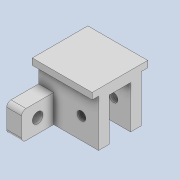
# Autodesk Inventor part: 10-03-025
Saved by Autodesk Inventor 2020 (Build 240168000, 168)
## iProperties
Created: 2019-11-02
Part Number: 10-03-025
Material: Generic
Document SubType Name: Modeling
Designer: iuliu
Density: 1 g/cm^3
Appearance: Default
Description: Intinzator Y
Mass: 10.4136 g
Surface Area: 53.1849 cm^2
Volume: 10.4136 cm^3
Author: iuliu
Subject: 036
Autodesk Inventor part; units mm, degrees
ref_plane "YZ Plane" through (0, 0, 0) normal (1, 0, 0) x (0, 1, 0)
ref_plane "XZ Plane" through (0, 0, 0) normal (0, 1, 0) x (-1, 0, 0)
ref_plane "XY Plane" through (0, 0, 0) normal (0, 0, 1) x (1, 0, 0)
sketch "Sketch7" plane through (0, 0, 0) normal (1, 0, 0) x (0, 0, -1)
  line L0 (10, -2.5) -> (-10, -2.5)
  line L1 (-10, -2.5) -> (-10, 22.5)
  line L2 (-10, 22.5) -> (10, 22.5)
  line L3 (10, 22.5) -> (10, -2.5)
  line L4 (13, 19.5) -> (10, 19.5)
  line L5 (10, 19.5) -> (10, 22.5)
  line L6 (10, 22.5) -> (13, 22.5)
  line L7 (13, 22.5) -> (13, 19.5)
  line L8 (-10, 19.5) -> (-13, 19.5)
  line L9 (-13, 19.5) -> (-13, 22.5)
  line L10 (-13, 22.5) -> (-10, 22.5)
  line L11 (-10, 22.5) -> (-10, 19.5)
  point P0 (0, -2.5)
  point P1 (0, 22.5)
  dimension "d26" = 20
  dimension "d27" = 25
  dimension "d30" = 3
  dimension "d31" = 3
  dimension "d32" = 3
  dimension "d33" = 3
  dimension "d72" = 0
  constraints: 24 end point, 6 parallel, 3 horizontal, 3 perpendicular, 1 collinear, 1 midpoint, 1 point on line
  measures "d26" distance between parallel lines of L1 L3
  measures "d27" distance of L2.end L0.start
  measures "d30" distance of L6.end L4.start
  measures "d31" distance of L4.start L4.end
  measures "d32" distance of L8.start L8.end
  measures "d33" distance of L8.end L9.end
  measures "d72" distance from line of point (0, -2.5) L0
extrude "Extrusion4" add sketch "Sketch7" along normal blind 28
sketch "Sketch15" plane through (0, -2.5, -10) normal (0, 0, -1) x (-1, 0, 0)
  line L0 (0, 0) -> (-28, 0) projected
  line L1 (-28, 0) -> (-28, 22) projected
  point P0 (0, 2.5)
  point P1 (-20, 10)
  dimension "d78" = 8
  dimension "d98" = 10
  measures "d78" distance from line of L1 point (-20, 10)
  measures "d98" distance from line of L0 point (-20, 10)
sketch "Sketch14" plane through (0, -2.5, -10) normal (0, -1, 0) x (1, 0, 0)
  line L0 (7, 15) -> (28, 15)
  line L1 (28, 15) -> (28, 5)
  line L2 (28, 5) -> (7, 5)
  line L3 (7, 5) -> (7, 15)
  line L4 (28, 20) -> (28, 0) projected
  point P0 (0, 10)
  point P1 (28, 10)
  point P2 (28, 10)
  dimension "d73" = 10
  dimension "d74" = 21
  constraints: 8 end point, 2 midpoint, 2 parallel, 1 coincident, 1 collinear, 1 horizontal, 1 perpendicular
  measures "d73" distance of L0.end L1.end
  measures "d74" distance of L0.start L0.end
extrude "Extrusion8" cut sketch "Sketch14" against normal blind 20
hole "Hole6" at (20, 7.5, -10) direction (0, 0, 1) diameter 4.134 end through all thread size "M5x0.8" class "6H" standard "ISO Metric profile"
sketch "Sketch16" plane through (0, 0, 0) normal (-1, 0, 0) x (0, 0, 1)
  line L0 (25, -2.5) -> (-25, -2.5)
  line L1 (-25, -2.5) -> (-25, 10.5)
  line L2 (-25, 10.5) -> (25, 10.5)
  line L3 (25, 10.5) -> (25, -2.5)
  line L4 (10, -2.5) -> (-10, -2.5) projected
  line L5 (-10, -2.5) -> (-10, 19.5) projected
  line L6 (10, 19.5) -> (10, -2.5) projected
  circle A0 centre (17.5, 4) radius 2.5
  circle A1 centre (-17.5, 4) radius 2.5
  point P0 (0, 0)
  point P1 (25, 4)
  point P2 (-10, -2.5)
  point P3 (-10, 10.5)
  point P4 (10, 10.5)
  point P5 (10, -2.5)
  dimension "d86" = 15
  dimension "d88" = 15
  dimension "d89" = 13
  dimension "d90" = 5
  dimension "d91" = 7.5
  dimension "d92" = 7.5
  constraints: 8 end point, 2 centre point, 2 horizontal alignment, 2 parallel, 1 collinear, 1 equal radius, 1 horizontal, 1 midpoint, 1 perpendicular
  measures "d86" distance between parallel lines of L5 L1
  measures "d88" distance between parallel lines of L6 L3
  measures "d89" distance of L2.end L0.start
  measures "d90" diameter of A0
  measures "d91" distance from line of A0.centre L3
  measures "d92" distance from line of L1 A1.centre
extrude "Extrusion9" add sketch "Sketch16" against normal blind 7 contours L0 L6 L2 L3 | L0 L1 L2 L5
fillet "Fillet1" radius 2 4 edges at (3.5, -2.5, -25) (3.5, 10.5, -25) (3.5, -2.5, 25) (3.5, 10.5, 25)
sketch "Sketch17" plane through (0, 0, 0) normal (-1, 0, 0) x (0, 0, 1)
  circle A0 centre (17.5, 4) radius 4.5
  circle A1 centre (-17.5, 4) radius 4.5
  circle A2 centre (-17.5, 4) radius 2.5 projected
  circle A3 centre (17.5, 4) radius 2.5 projected
  point P0 (0, 0)
  dimension "d99" = 9
  constraints: 2 centre point, 2 concentric, 1 equal radius
  measures "d99" diameter of A0
extrude "Extrusion10" cut sketch "Sketch17" against normal blind 2
equation "\"d88\" = d86"
equation "\"d91\" = 0.5 * d88"
equation "\"d92\" = d91"
body "Solid1"
